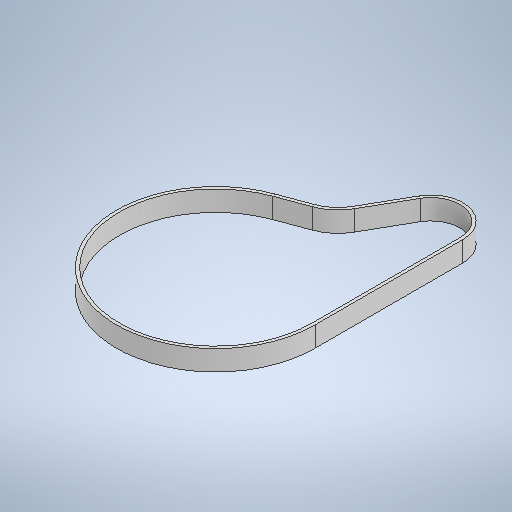
# Autodesk Inventor part: 50-01-001
Saved by Autodesk Inventor 2025.2 (Build 292293000, 293)
## iProperties
Created: 2024-11-29
Part Number: 50-01-001
Material: Generic
Document SubType Name: Modeling
Designer: Zvonko.Gabric
Density: 1 g/cm^3
Appearance: Default
Author: Zvonko.Gabric
Autodesk Inventor part; units mm, degrees
ref_plane "YZ Plane" through (0, 0, 0) normal (1, 0, 0) x (0, 1, 0)
ref_plane "XZ Plane" through (0, 0, 0) normal (0, 1, 0) x (-1, 0, 0)
ref_plane "XY Plane" through (0, 0, 0) normal (0, 0, 1) x (1, 0, 0)
sketch "Sketch1" plane through (0, 0, 0) normal (0, 1, 0) x (-1, 0, 0)
  line L0 (70.8919, 46.3756) -> (99.3426, 56.8576)
  line L1 (24.7543, -14.1235) -> (48.4088, 27.336)
  line L2 (-28.5, 146) -> (-28.5, 0)
  line L3 (51.0145, 25.8493) -> (27.3601, -15.6101)
  line L4 (100.3797, 54.0426) -> (71.929, 43.5606)
  line L5 (-31.5, 0) -> (-31.5, 146)
  arc A0 (99.3426, 56.8576) -> (-28.5, 146) centre (66.5, 146) ccw
  arc A1 (70.8919, 46.3756) -> (48.4088, 27.336) centre (85.7575, 6.0269) ccw
  arc A2 (-28.5, 0) -> (24.7543, -14.1235) centre (0, 0) ccw
  arc A3 (-31.5, 0) -> (27.3601, -15.6101) centre (0, 0) ccw
  arc A4 (71.929, 43.5606) -> (51.0145, 25.8493) centre (85.7575, 6.0269) ccw
  arc A5 (100.3797, 54.0426) -> (-31.5, 146) centre (66.5, 146) ccw
  dimension "d0" = 95
  dimension "d1" = 40
  dimension "d2" = 28.5
  dimension "d3" = 31.5
  dimension "d4" = 146
  dimension "d5" = 146
  dimension "d6" = 98
  dimension "d7" = 95
  dimension "d8" = 146
  dimension "d9" = 66.5
  dimension "d10" = 47.7328
  dimension "d11" = 53.2544
  dimension "d12" = 43
  dimension "d13" = 58.8601
  dimension "d14" = 47.7328
  dimension "d15" = 91.9574
  dimension "d16" = 139.9731
  dimension "d17" = 85.7575
  dimension "d18" = 150.293
  dimension "d19" = 0
  dimension "d20" = 0
  constraints: 12 end point, 12 point on circle, 6 centre point
  measures "d0" radius of A0
  measures "d1" radius of A4
  measures "d2" radius of A2
  measures "d3" radius of A3
  measures "d4" distance of L2.start L2.end
  measures "d5" distance of L5.start L5.end
  measures "d6" radius of A5
  measures "d7" distance from line of A0.centre L2
  measures "d8" vertical distance of A0.centre A2.centre
  measures "d9" horizontal distance of A0.centre A2.centre
  measures "d10" distance of L3.start L3.end
  measures "d11" horizontal distance of L2.end L1.start
  measures "d12" radius of A1
  measures "d13" horizontal distance of L5.start L3.end
  measures "d14" distance of L1.start L1.end
  measures "d15" vertical distance of L4.start L5.end
  measures "d16" vertical distance of A0.centre A1.centre
  measures "d17" horizontal distance of A2.centre A1.centre
  measures "d19" distance of point (0, 0) A2.centre
  measures "d20" distance of point (0, 0) A2.centre
extrude "Extrusion1" add sketch "Sketch1" along normal blind 20
body "Solid1"
